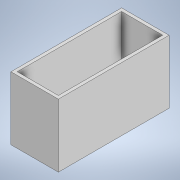
# Autodesk Inventor part: servo housing
Saved by Autodesk Inventor 2022 (Build 260153000, 153)
## iProperties
Created: 2022-01-29
Part Number: servo housing
Material: Generic
Document SubType Name: Modeling
Designer: peter
Density: 1 g/cm^3
Appearance: Default
Author: peter
Autodesk Inventor part; units mm, degrees
ref_plane "YZ Plane" through (0, 0, 0) normal (1, 0, 0) x (0, 1, 0)
ref_plane "XZ Plane" through (0, 0, 0) normal (0, 1, 0) x (-1, 0, 0)
ref_plane "XY Plane" through (0, 0, 0) normal (0, 0, 1) x (1, 0, 0)
sketch "Sketch1" plane through (0, 0, 0) normal (0, 1, 0) x (-1, 0, 0)
  line L0 (7.5, 17.5) -> (-7.5, 17.5)
  line L1 (-7.5, 17.5) -> (-7.5, -17.5)
  line L2 (-7.5, -17.5) -> (7.5, -17.5)
  line L3 (7.5, -17.5) -> (7.5, 17.5)
  line L4 (7.5, 17.5) -> (-7.5, -17.5) construction
  line L5 (-7.5, 17.5) -> (7.5, -17.5) construction
  point P0 (0, 0)
  dimension "d0" = 35
  dimension "d1" = 15
  constraints: 12 end point, 2 midpoint, 2 parallel, 1 horizontal, 1 perpendicular
  measures "d0" distance of L2.end L0.start
  measures "d1" distance of L0.start L0.end
extrude "Extrusion1" add sketch "Sketch1" along normal blind 20
shell "Shell1" thickness 1 removed faces 1 at (2.5, 20, -5.8333)
body "Solid1"
